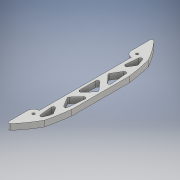
# Autodesk Inventor part: ガイド横上
Saved by Autodesk Inventor 2018.3 (Build 223284000, 284)
## iProperties
Created: 2019-04-06
Part Number: ガイド横上
Material: 一般
Document SubType Name: Modeling
Designer: shun2
Density: 1 g/cm^3
Appearance: 既定
Author: shun2
Autodesk Inventor part; units mm, degrees
ref_plane "YZ Plane" through (0, 0, 0) normal (1, 0, 0) x (0, 1, 0)
ref_plane "XZ Plane" through (0, 0, 0) normal (0, 1, 0) x (-1, 0, 0)
ref_plane "XY Plane" through (0, 0, 0) normal (0, 0, 1) x (1, 0, 0)
sketch "スケッチ1" plane through (0, 0, 0) normal (0, 0, 1) x (1, 0, 0)
  arc A0 (0, 5.1191) -> (3.497, 3.7928) centre (2, 5.1191) ccw
  arc A1 (3.497, 3.7928) -> (20.2574, 27.638) centre (-93.8083, 90) ccw
  arc A2 (20.2574, 27.638) -> (25.3494, 55.5364) centre (-242.442, 90) ccw
  line L0 (25.3494, 55.5364) -> (25.3494, 124.4636)
  arc A3 (25.3494, 124.4636) -> (20.2574, 152.362) centre (-242.442, 90) ccw
  arc A4 (20.2574, 152.362) -> (3.497, 176.2072) centre (-93.8083, 90) ccw
  arc A5 (3.497, 176.2072) -> (0, 174.8809) centre (2, 174.8809) ccw
  line L1 (0, 174.8809) -> (0, 152.362)
  arc A6 (0, 152.362) -> (7, 145.362) centre (7, 152.362) ccw
  line L2 (7, 145.362) -> (7, 109.815)
  line L3 (7, 80.815) -> (7, 34.638)
  arc A7 (7, 34.638) -> (0, 27.638) centre (7, 27.638) ccw
  line L4 (0, 27.638) -> (0, 5.1191)
  arc A8 (20.8277, 125.2984) -> (17.1291, 126.1497) centre (18.8368, 125.1086) ccw
  line L5 (20.8277, 125.2984) -> (22.6836, 105.8325)
  arc A9 (19.2111, 104.2992) -> (22.6836, 105.8325) centre (20.6926, 105.6427) ccw
  line L6 (19.2111, 104.2992) -> (11.0046, 113.3481)
  arc A10 (10.7784, 115.7327) -> (11.0046, 113.3481) centre (12.4861, 114.6917) ccw
  line L7 (10.7784, 115.7327) -> (17.1291, 126.1497)
  arc A11 (18.8075, 140.2289) -> (18.979, 141.9846) centre (17.1068, 141.2812) ccw
  line L8 (18.8075, 140.2289) -> (14.4979, 133.2642)
  arc A12 (10.8061, 134.5052) -> (14.4979, 133.2642) centre (12.7972, 134.3166) ccw
  line L9 (10.8061, 134.5052) -> (12.2009, 149.2292)
  arc A13 (16.0642, 149.7439) -> (12.2009, 149.2292) centre (14.192, 149.0405) ccw
  line L10 (16.0642, 149.7439) -> (18.979, 141.9846)
  arc A14 (14.4979, 46.7358) -> (10.8061, 45.4948) centre (12.7972, 45.6834) ccw
  line L11 (14.4979, 46.7358) -> (18.8075, 39.7711)
  arc A15 (18.979, 38.0154) -> (18.8075, 39.7711) centre (17.1068, 38.7188) ccw
  line L12 (18.979, 38.0154) -> (16.0642, 30.2561)
  arc A16 (12.2009, 30.7708) -> (16.0642, 30.2561) centre (14.192, 30.9595) ccw
  line L13 (12.2009, 30.7708) -> (10.8061, 45.4948)
  arc A17 (11.0046, 66.6519) -> (10.7784, 64.2673) centre (12.4861, 65.3083) ccw
  line L14 (11.0046, 66.6519) -> (19.2111, 75.7008)
  arc A18 (22.6836, 74.1675) -> (19.2111, 75.7008) centre (20.6926, 74.3573) ccw
  line L15 (22.6836, 74.1675) -> (20.8277, 54.7016)
  arc A19 (17.1291, 53.8503) -> (20.8277, 54.7016) centre (18.8368, 54.8914) ccw
  line L16 (17.1291, 53.8503) -> (10.7784, 64.2673)
  arc A20 (13.4987, 101.0407) -> (10, 99.7163) centre (12, 99.7163) ccw
  line L17 (13.4987, 101.0407) -> (22.0846, 91.3243)
  arc A21 (22.0846, 88.6757) -> (22.0846, 91.3243) centre (20.5859, 90) ccw
  line L18 (22.0846, 88.6757) -> (13.4987, 78.9593)
  arc A22 (10, 80.2837) -> (13.4987, 78.9593) centre (12, 80.2837) ccw
  line L19 (10, 80.2837) -> (10, 99.7163)
  circle A23 centre (7, 152.362) radius 1.5
  circle A24 centre (7, 27.638) radius 1.5
  line L20 (7, 109.815) -> (7, 80.815)
  point P0 (0, 0)
  point P1 (0, 0)
  constraints: 46 point on circle, 42 end point, 25 centre point, 1 vertical
extrude "押し出し1" add sketch "スケッチ1" along normal blind 7
